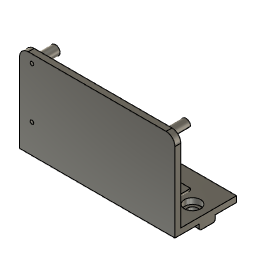
Gantry Mount v6 (Autodesk Fusion 360 design; units mm, degrees)
Autodesk Fusion 360 part; units mm, degrees
note: some values were not read from the file. Chosen so that the rebuilt part matches the saved one: which bodies a step acts on; which face or edge a step refers to. Set by a fixed rule: which sketch regions a step uses.
sketch "Sketch1" plane through (0, 0, 0) normal (0, 0, 1) x (1, 0, 0)
  line L0 (0, 0) -> (53, 0)
  line L1 (53, 0) -> (53, 20)
  line L2 (53, 20) -> (0, 20)
  line L3 (0, 20) -> (0, 0)
  line L4 (0, 10) -> (53, 10) construction
  line L5 (0, 7.25) -> (53, 7.25)
  line L6 (0, 12.75) -> (53, 12.75)
  circle A0 centre (5, 10) radius 1.75
  line L7 (26.5, 0) -> (26.5, 20) construction
  circle A1 centre (48, 10) radius 1.75
  circle A2 centre (5, 10) radius 2.75
  circle A3 centre (48, 10) radius 2.75
  dimension "d1" = 53
  dimension "d2" = 20
  dimension "d4" = 3.5
  dimension "d5" = 5
  dimension "d23" = 5.5
  dimension "d54" = 7.25
  dimension "d55" = 7.25
  constraint horizontal L0
  constraint vertical L1
  constraint horizontal L2
  constraint vertical L3
  constraint coincident L0.start L3.end
  constraint midpoint L3 L4.start
  constraint midpoint L1 L4.end
  constraint coincident L3 L5.start
  constraint coincident L1 L5.end
  constraint perpendicular L1 L5
  constraint symmetric L4 L5.start L6.start
  constraint symmetric L4 L5.end L6.end
  constraint coincident L4 A0.centre
  constraint midpoint L0 L7.start
  constraint midpoint L2 L7.end
  constraint symmetric A0 L7 A1
  constraint concentric A0 A2
  constraint symmetric L7 A2 A3
  measures "d1" distance of L0.start L0.end
  measures "d2" distance of L0.start L2.end
  measures "d4" diameter of A0
  measures "d5" distance of L3 A0.centre
  measures "d23" diameter of A2
  measures "d54" distance of L2 L6
  measures "d55" distance of L0 L5
sketch "Sketch2" plane through (0, 0, 0) normal (0, 1, 0) x (1, 0, 0)
  line L0 (0, 0) -> (53, 0)
  line L1 (53, 0) -> (53, -30)
  line L2 (0, -30) -> (0, 0)
  line L3 (0, -2) -> (53, -2)
  line L4 (0, 0) -> (53, 0)
  circle A0 centre (4.25, -27.15) radius 0.6
  circle A1 centre (4.25, -27.15) radius 1.6
  line L5 (0, -18.5) -> (53, -18.5) construction
  circle A2 centre (4.25, -9.85) radius 0.6
  line L6 (26.5, -30) -> (26.5, -2) construction
  line L7 (53, -30) -> (26.5, -30)
  line L8 (26.5, -30) -> (0, -30)
  line L9 (4.25, -27.15) -> (4.25, -1) construction
  circle A3 centre (4.25, -9.85) radius 1.6
  line L10 (48.75, -27.65) -> (48.75, -1) construction
  line L11 (4.25, -9.85) -> (61, -9.85) construction
  line L12 (4.25, -27.15) -> (55.5531, -27.15) construction
  line L13 (48.75, -9.35) -> (50.35, -9.35)
  line L14 (48.75, -9.35) -> (47.15, -9.35)
  arc A4 (50.35, -9.35) -> (47.15, -9.35) centre (48.75, -9.35) ccw
  line L15 (48.75, -27.65) -> (50.35, -27.65)
  line L16 (48.75, -27.65) -> (47.15, -27.65)
  arc A5 (47.15, -27.65) -> (50.35, -27.65) centre (48.75, -27.65) ccw
  point P0 (0, -30)
  point P1 (48.75, -27.15)
  point P2 (48.75, -4.35)
  dimension "d6" = 30
  dimension "d7" = 2
  dimension "d10" = 1
  dimension "d11" = 11.5
  dimension "d12" = 16.5
  dimension "d24" = 53
  dimension "d31" = 2.85
  dimension "d39" = 17.3
  dimension "d40" = 1
  dimension "d41" = 3.2
  dimension "d42" = 3.2
  dimension "d43" = 3.2
  dimension "d46" = 3.2
  dimension "d49" = 44.5
  dimension "d61" = 2.35
  dimension "d62" = 18.3
  constraint horizontal L0
  constraint vertical L1
  constraint horizontal L7
  constraint vertical L2
  constraint coincident L0.start L2.end
  constraint coincident L2 L3.start
  constraint coincident L1 L3.end
  constraint perpendicular L1 L3
  constraint concentric A0 A1
  constraint coincident L2 L5.start
  constraint coincident L1 L5.end
  constraint perpendicular L1 L5
  constraint midpoint L3 L6.end
  constraint coincident L6.start L7
  constraint coincident P0 L7
  constraint coincident P0 L2
  constraint coincident P0 L2.start
  constraint coincident A0.centre A1.centre
  constraint perpendicular L3 L9
  constraint concentric A2 A3
  constraint perpendicular L3 L10
  constraint coincident A2.centre A3.centre
  constraint perpendicular L1 L11
  constraint coincident L10.start L15.start
  constraint coincident L10 P1
  constraint coincident L12 P1
  constraint coincident L13.start L14.start
  constraint perpendicular L10 L13
  constraint parallel L13 L14
  constraint perpendicular L10 L15
  constraint parallel L15 L16
  measures "d6" distance of L0.start P0
  measures "d7" distance of L3 L4
  measures "d10" distance of A0 A1
  measures "d11" distance of L5 L7
  measures "d12" distance of L3 L5
  measures "d24" distance of L0.start L0.end
  measures "d31" distance of A0.centre L8
  measures "d39" distance of A0.centre A2.centre
  measures "d40" distance of A2 A3
  measures "d41" diameter of A1
  measures "d42" diameter of A3
  measures "d43" diameter of A4
  measures "d46" diameter of A5
  measures "d49" distance of A0.centre P1
  measures "d61" distance of L7 L10.start
  measures "d62" distance of L13.start L10.start
extrude "Extrude1" add sketch "Sketch2" along normal blind 8 contours A1 | A3 makes body 1 at (5.848, 5.3333, 9.9298) makes body 2 at (5.848, 5.3333, 27.2298)
extrude "Extrude2" add sketch "Sketch2" along normal blind 2 contours L1 L2 L3 L7 L8 | A2 | A3 | L13 L14 A4 | L15 L16 A5 bodies 1 2
extrude "Extrude3" add sketch "Sketch1" along normal blind 2 bodies 1
extrude "Extrude4" add sketch "Sketch1" against normal blind 2 contours L3 L5 L6 A2 | L1 L5 L6 A3 | L5 L6 A2 A3 | A2 | A3 bodies 1
chamfer "Chamfer1" distance 0.5 angle 45 2 edges at (26.5, 12.75, -2) (26.5, 7.25, -2) on bodies 1
extrude "Extrude5" add sketch "Sketch1" along normal blind 2.5 contours A2 | A3 bodies 1
extrude "Extrude6" cut 2 faces at (7.3999, 10.2236, 2.5) (50.3999, 10.2236, 2.5) along direction (0, 0, -1) blind 2.5 on bodies 1 bodies 1
extrude "Extrude7" cut 2 faces at (5.5085, 8, 27.2593) (5.5085, 8, 9.9593) along direction (0, -1, 0) blind 1 on bodies 1 bodies 1
extrude "Extrude8" cut 1 faces at (37.2596, 2, 14.1072) along direction (0, -1, 0) blind 1 on bodies 1 bodies 1
extrude "Extrude9" cut 1 faces at (19.9049, 17.3833, 2) along direction (0, 0, -1) blind 1 on bodies 1 bodies 1
extrude "Extrude10" add sketch "Sketch2" along normal blind 5 contours L13 L14 A4 | L15 L16 A5 bodies 1
extrude "Extrude11" add 2 faces at (48.4175, 5, 28.3814) (49.0825, 5, 8.6186) along direction (0, 1, 0) blind 2 on bodies 1 bodies 1
extrude "Extrude12" add 1 faces at (36.9338, 0, 18.9711) along direction (0, -1, 0) blind 1 on bodies 1 bodies 1
extrude "Extrude13" add 1 faces at (19.9049, 17.3833, 1) along direction (0, 0, 1) blind 1 on bodies 1 bodies 1
extrude "Extrude14" cut 1 faces at (4.3231, 2, 10.0362) along direction (0, -1, 0) blind 3 on bodies 1 bodies 1
fillet "Fillet1" radius 3 2 edges at (0, 0, 30) (53, 0, 30) on bodies 1
chamfer "Chamfer2" [rolled back] distance 3
